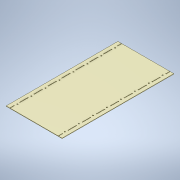
# Autodesk Inventor part: top_bottom_layer_3mm
Saved by Autodesk Inventor 2021 (Build 250183000, 183)
## iProperties
Created: 2021-01-27
Part Number: top_bottom_layer_3mm
Material: Acrylic
Document SubType Name: Modeling
Designer: abij996
Density: 1.188 g/cm^3
Appearance: Smooth - Ash
Author: abij996
Autodesk Inventor part; units mm, degrees
ref_plane "YZ Plane" through (0, 0, 0) normal (1, 0, 0) x (0, 1, 0)
ref_plane "XZ Plane" through (0, 0, 0) normal (0, 1, 0) x (-1, 0, 0)
ref_plane "XY Plane" through (0, 0, 0) normal (0, 0, 1) x (1, 0, 0)
sketch "Sketch2" plane through (0, 0, 0) normal (0, 1, 0) x (-1, 0, 0)
  line L0 (238.7833, 367.5648) -> (-161.2167, 367.5648)
  line L1 (-161.2167, 367.5648) -> (-161.2167, -432.4352)
  line L2 (-161.2167, -432.4352) -> (238.7833, -432.4352)
  line L3 (238.7833, -432.4352) -> (238.7833, 367.5648)
  circle A0 centre (208.7833, 217.5631) radius 4
  circle A1 centre (208.7833, 317.5673) radius 4
  circle A2 centre (208.7833, -382.4352) radius 4
  circle A3 centre (208.7833, -283.981) radius 4
  circle A4 centre (208.7833, -183.981) radius 4
  circle A5 centre (208.7833, -83.981) radius 4
  circle A6 centre (208.7833, 16.019) radius 4
  circle A7 centre (208.7833, 116.019) radius 4
  line L4 (38.7833, -432.4352) -> (38.7833, 367.5648) construction
  line L5 (208.7833, 217.5631) -> (208.7833, 317.5673) construction
  line L6 (208.7833, 317.5673) -> (208.7833, 367.5648) construction
  line L7 (208.7833, -382.4352) -> (208.7833, -432.4352) construction
  line L8 (208.7833, -382.4352) -> (208.7833, 217.5631) construction
  line L9 (213.7833, -263.981) -> (210.2833, -263.981)
  line L10 (210.2833, -263.981) -> (210.2833, -203.981)
  line L11 (210.2833, -203.981) -> (213.7833, -203.981)
  line L12 (213.7833, -203.981) -> (213.7833, -263.981)
  line L13 (213.7833, 196.019) -> (210.2833, 196.019)
  line L14 (210.2833, 196.019) -> (210.2833, 136.019)
  line L15 (210.2833, 136.019) -> (213.7833, 136.019)
  line L16 (213.7833, 136.019) -> (213.7833, 196.019)
  line L17 (213.7833, -3.981) -> (210.2833, -3.981)
  line L18 (210.2833, -3.981) -> (210.2833, -63.981)
  line L19 (210.2833, -63.981) -> (213.7833, -63.981)
  line L20 (213.7833, -63.981) -> (213.7833, -3.981)
  line L21 (213.7833, 34.2998) -> (210.2833, 34.2998)
  line L22 (210.2833, 34.2998) -> (210.2833, 94.2998)
  line L23 (210.2833, 94.2998) -> (213.7833, 94.2998)
  line L24 (213.7833, 94.2998) -> (213.7833, 34.2998)
  line L25 (213.7833, -163.981) -> (210.2833, -163.981)
  line L26 (210.2833, -163.981) -> (210.2833, -103.981)
  line L27 (210.2833, -103.981) -> (213.7833, -103.981)
  line L28 (213.7833, -103.981) -> (213.7833, -163.981)
  line L29 (213.7833, -362.4352) -> (210.2833, -362.4352)
  line L30 (210.2833, -362.4352) -> (210.2833, -302.4352)
  line L31 (210.2833, -302.4352) -> (213.7833, -302.4352)
  line L32 (213.7833, -302.4352) -> (213.7833, -362.4352)
  line L33 (210.2833, 237.5631) -> (213.7833, 237.5631)
  line L34 (213.7833, 237.5631) -> (213.7833, 297.5631)
  line L35 (213.7833, 297.5631) -> (210.2833, 297.5631)
  line L36 (210.2833, 297.5631) -> (210.2833, 237.5631)
  line L37 (210.2833, 337.5673) -> (213.7833, 337.5673)
  line L38 (213.7833, 337.5673) -> (213.7833, 367.5648)
  line L39 (213.7833, 367.5648) -> (210.2833, 367.5648)
  line L40 (210.2833, 367.5648) -> (210.2833, 337.5673)
  line L41 (213.7833, -432.4352) -> (210.2833, -432.4352)
  line L42 (210.2833, -432.4352) -> (210.2833, -402.4352)
  line L43 (210.2833, -402.4352) -> (213.7833, -402.4352)
  line L44 (213.7833, -402.4352) -> (213.7833, -432.4352)
  circle A8 centre (-131.2167, 217.5631) radius 4
  circle A9 centre (-131.2167, 317.5673) radius 4
  circle A10 centre (-131.2167, -382.4352) radius 4
  circle A11 centre (-131.2167, -283.981) radius 4
  circle A12 centre (-131.2167, -183.981) radius 4
  circle A13 centre (-131.2167, -83.981) radius 4
  circle A14 centre (-131.2167, 16.019) radius 4
  circle A15 centre (-131.2167, 116.019) radius 4
  line L45 (-131.2167, 217.5631) -> (-131.2167, 317.5673) construction
  line L46 (-131.2167, 317.5673) -> (-131.2167, 367.5648) construction
  line L47 (-131.2167, -382.4352) -> (-131.2167, -432.4352) construction
  line L48 (-131.2167, -382.4352) -> (-131.2167, 217.5631) construction
  line L49 (-136.2167, -263.981) -> (-132.7167, -263.981)
  line L50 (-132.7167, -263.981) -> (-132.7167, -203.981)
  line L51 (-132.7167, -203.981) -> (-136.2167, -203.981)
  line L52 (-136.2167, -203.981) -> (-136.2167, -263.981)
  line L53 (-136.2167, 196.019) -> (-132.7167, 196.019)
  line L54 (-132.7167, 196.019) -> (-132.7167, 136.019)
  line L55 (-132.7167, 136.019) -> (-136.2167, 136.019)
  line L56 (-136.2167, 136.019) -> (-136.2167, 196.019)
  line L57 (-136.2167, -3.981) -> (-132.7167, -3.981)
  line L58 (-132.7167, -3.981) -> (-132.7167, -63.981)
  line L59 (-132.7167, -63.981) -> (-136.2167, -63.981)
  line L60 (-136.2167, -63.981) -> (-136.2167, -3.981)
  line L61 (-136.2167, 34.2998) -> (-132.7167, 34.2998)
  line L62 (-132.7167, 34.2998) -> (-132.7167, 94.2998)
  line L63 (-132.7167, 94.2998) -> (-136.2167, 94.2998)
  line L64 (-136.2167, 94.2998) -> (-136.2167, 34.2998)
  line L65 (-136.2167, -163.981) -> (-132.7167, -163.981)
  line L66 (-132.7167, -163.981) -> (-132.7167, -103.981)
  line L67 (-132.7167, -103.981) -> (-136.2167, -103.981)
  line L68 (-136.2167, -103.981) -> (-136.2167, -163.981)
  line L69 (-136.2167, -362.4352) -> (-132.7167, -362.4352)
  line L70 (-132.7167, -362.4352) -> (-132.7167, -302.4352)
  line L71 (-132.7167, -302.4352) -> (-136.2167, -302.4352)
  line L72 (-136.2167, -302.4352) -> (-136.2167, -362.4352)
  line L73 (-132.7167, 237.5631) -> (-136.2167, 237.5631)
  line L74 (-136.2167, 237.5631) -> (-136.2167, 297.5631)
  line L75 (-136.2167, 297.5631) -> (-132.7167, 297.5631)
  line L76 (-132.7167, 297.5631) -> (-132.7167, 237.5631)
  line L77 (-132.7167, 337.5673) -> (-136.2167, 337.5673)
  line L78 (-136.2167, 337.5673) -> (-136.2167, 367.5648)
  line L79 (-132.7167, 367.5648) -> (-132.7167, 337.5673)
  line L80 (-132.7167, -432.4352) -> (-132.7167, -402.4352)
  line L81 (-132.7167, -402.4352) -> (-136.2167, -402.4352)
  line L82 (-136.2167, -402.4352) -> (-136.2167, -432.4352)
  point P0 (0, 0)
  dimension "d46" = 800
  dimension "d47" = 400
  dimension "d67" = 50
  dimension "d90" = 3.5
  dimension "d91" = 60
  dimension "d93" = 25
  dimension "d94" = 20
  dimension "d95" = 3.5
  dimension "d96" = 3.5
  dimension "d97" = 25
  dimension "d98" = 20
  dimension "d99" = 20
  dimension "d100" = 60
  dimension "d101" = 60
  dimension "d102" = 3.5
  dimension "d103" = 25
  dimension "d104" = 18.2808
  dimension "d105" = 60
  dimension "d106" = 25
  dimension "d107" = 3.5
  dimension "d108" = 20
  dimension "d109" = 60
  dimension "d110" = 3.5
  dimension "d111" = 60
  dimension "d112" = 20
  dimension "d113" = 25
  dimension "d114" = 3.5
  dimension "d115" = 25
  dimension "d116" = 20
  dimension "d117" = 60
  dimension "d118" = 3.5
  dimension "d119" = 25
  dimension "d120" = 20
  dimension "d121" = 3.5
  dimension "d123" = 25
  dimension "d124" = 20
  constraints: 166 end point, 46 symmetric about line, 20 parallel, 16 centre point, 10 horizontal, 10 perpendicular, 10 point on line, 2 midpoint, 1 collinear, 1 vertical, 16 other
  measures "d46" distance of L2.end L0.start
  measures "d47" distance of L0.start L0.end
  measures "d67" distance from line of L2 L7.start
  measures "d90" distance between parallel lines of L12 L10
  measures "d91" distance of L9.end L10.end
  measures "d93" distance between parallel lines of L3 L12
  measures "d94" distance from line of A3.centre L9
  measures "d95" distance between parallel lines of L16 L14
  measures "d96" distance between parallel lines of L20 L18
  measures "d97" distance between parallel lines of L3 L20
  measures "d98" distance from line of L19 A5.centre
  measures "d99" distance from line of L15 A7.centre
  measures "d100" distance of L17.end L18.end
  measures "d101" distance of L13.end L14.end
  measures "d102" distance between parallel lines of L24 L22
  measures "d103" distance between parallel lines of L3 L24
  measures "d104" distance from line of A6.centre L21
  measures "d105" distance of L21.end L22.end
  measures "d106" distance between parallel lines of L3 L28
  measures "d107" distance between parallel lines of L28 L26
  measures "d108" distance from line of L25 A4.centre
  measures "d109" distance of L25.end L26.end
  measures "d110" distance between parallel lines of L32 L30
  measures "d111" distance of L29.end L30.end
  measures "d112" distance from line of L7.start L29
  measures "d113" distance between parallel lines of L3 L32
  measures "d114" distance between parallel lines of L34 L36
  measures "d115" distance between parallel lines of L3 L34
  measures "d116" distance from line of L5.start L33
  measures "d117" distance of L35.end L33.start
  measures "d118" distance between parallel lines of L40 L38
  measures "d119" distance between parallel lines of L3 L38
  measures "d120" distance from line of L37 L5.end
  measures "d121" distance between parallel lines of L44 L42
  measures "d123" distance between parallel lines of L3 L44
  measures "d124" distance from line of L43 L7.start
extrude "Extrusion7" add sketch "Sketch2" along normal blind 3 contours L3 L2 L44 L43 L42 L80 L81 L82 L1 L0 L78 L77 L79 L40 L37 L38
body "Solid7"
